Autodesk Fusion 360 part; units mm, degrees
(part 4 of 4)
extrude "Extrusão23" cut sketch "Esboço21" against normal blind 1 contours S0 S1 S2 S3 L28 L29 S4 L30 L31 S5 S6 S7 S8 S9 S10 S11 S12 S13 S14 S15 S16 S17 S18 L32 L33 S19 L34 L35 S20 S21 S22 S23 S24 S25 S26 S27 S28 S29 S30 S31 S32 S33 S34 S35 S36 L36 L37 S37 S38 S39 S40 S41 S42 S43 S44 S45 S46 S47 S48 S49 S50 S51 S52 S53 S54 S55 S56 S57 S58 S59 S60 S61 S62 S63 S64 S65 S66 S67 S68 S69 L38 L39 S70 S71 S72 S73 S74 S75 S76 S77 S78 S79 S80 S81 S82 L40 L41 S83 S84 S85 L42 L43 S86 S87 S88 S89 S90 S91 S92 S93 L44 L45 S94 L46 L47 S95 S96 S97 S98 S99 S100 L48 L49 S101 S102 S103 S104 S105 S106 S107 | S248 S249 S250 S251 S252 S253 S254 S255 S256 S257 S258 S259 S260 S261 S262 S263 S264 S265 S266 S267 S268 S269 S270 S271 S272 S273 S274 S275 S276 S277 S278 S279 S280 S281 S282 S283 S284 S285 S286 S287 S288 S289 S290 S291 S292 | S311 S312 S313 S314 S315 S316 S317 | S324 S325 S326 S327 S328 S329 S330 S331 S332 S333 S334 S335 S336 S337 L62 L63 S338 S339 S340 S341 S342 S343 S344 S345 S346 S347 S348 S349 S350 S351 S352 S353 S354 S355 S356 S357 S358 S359 S360 S361 S362 S363 S364 S365 S366 S367 S368 S369 S370 S371 L64 L65 S372 S373 L66 L67 S374 S375 S376 S377 S378 S379 S380 S381 S382 S383 S384 S385 S386 L68 L69 S387 L70 L71 S388 S389 S390 S391 S392 S393 S394 S395 S396 S397 S398 S399 S400 S401 S402 S403 S404 S405 S406 S407 S408 S409 S410 S411 S412 S413 S414 L72 L73 S415 S416 S417 S418 S419 S420 S421 S422 S423 S424 S425 S426 L74 L75 S427 S428 S429 S430 S431 S432 S433 S434 S435 S436 | S654 S655 S656 | S672 S673 S674 S675 S676 S677 L100 L101 L102 L103 S678 bodies 2
sketch "Esboço22" plane through (0, 0, 24.51) normal (0, 0, -1) x (1, 0, 0)
  spline S0 degree 3 poles (210.2876, 111.6079) (210.4619, 111.38) (210.6257, 111.1299) (210.7764, 110.864) knots 0 0 0 0 0.232069 0.232069 0.232069 0.232069
  line L0 (210.7764, 110.864) -> (215.399, 110.864)
  line L1 (215.399, 110.864) -> (215.399, 125.864)
  line L2 (215.399, 125.864) -> (200.399, 125.864)
  line L3 (200.399, 125.864) -> (200.399, 112.7841)
  spline S1 degree 3 poles (200.399, 112.7841) (201.1419, 113.2879) (202.0331, 113.7075) (202.8355, 113.9186) knots 0.268953 0.268953 0.268953 0.268953 1 1 1 1
  spline S2 degree 3 poles (202.8355, 113.9186) (203.0738, 113.9836) (203.6226, 114.0703) (204.0631, 114.1136) knots 0 0 0 0 1 1 1 1
  spline S3 degree 3 poles (204.0631, 114.1136) (206.5038, 114.3663) (208.93, 113.3915) (210.2876, 111.6079) knots 0 0 0 0 1 1 1 1
  circle A0 centre (207.899, 118.364) radius 2.5
  line L4 (215.399, 121.8438) -> (200.399, 121.8438)
  line L5 (200.399, 121.8438) -> (200.399, 114.8842)
  line L6 (200.399, 114.8842) -> (215.399, 114.8842)
  line L7 (215.399, 114.8842) -> (215.399, 121.8438)
  line L8 (215.399, 121.8438) -> (200.399, 114.8842) construction
  line L9 (200.399, 121.8438) -> (215.399, 114.8842) construction
  line L10 (200.399, 114.8842) -> (215.399, 114.8842)
  line L11 (215.399, 114.8842) -> (215.399, 110.864)
  line L12 (215.399, 110.864) -> (200.399, 110.864)
  line L13 (200.399, 110.864) -> (200.399, 114.8842)
  point P0 (207.899, 118.364)
  constraint horizontal L4
  constraint perpendicular L4 L5
  constraint parallel L4 L6
  constraint parallel L5 L7
  constraint coincident L8 P0
  constraint coincident L9 P0
  constraint coincident L1 L4.start
  constraint coincident P0 A0.centre
  constraint horizontal L10
  constraint vertical L11
  constraint horizontal L12
  constraint vertical L13
  constraint coincident L0.end L1.start
extrude "Extrusão24" add sketch "Esboço22" along normal blind 1 contours S0 L0 L1 L3 S1 S2 S3 L6 L10 L11 L12 L13 | S0 S1 S2 S3 L12 L13 | L1 L2 L3 L4 bodies 2
sketch "Esboço23" plane through (269, 0, 0) normal (1, 0, 0) x (0, 1, 0)
  line L0 (-40.5, 23.51) -> (-140.5, 23.51)
  line L1 (-140.5, 23.51) -> (-140.5, 13.51)
  line L2 (-140.5, 13.51) -> (-40.5, 13.51)
  line L3 (-40.5, 13.51) -> (-40.5, 23.51)
  line L4 (-40.5, 23.51) -> (-51.0189, 13.51)
  constraint coincident L0.start L3.end
  constraint coincident L2 L4.end
extrude "Extrusão25" cut sketch "Esboço23" against normal blind 185 contours L2 L3 L4 bodies 2
sketch "Esboço24" plane through (271.5, 0, 0) normal (1, 0, 0) x (0, 1, 0)
  circle A0 centre (-90.5, 11.01) radius 7
  line L0 (-38, -11.49) -> (-38, 23.51)
  line L1 (-38, 23.51) -> (-143, 23.51)
  line L2 (-143, 23.51) -> (-143, -11.49)
  line L3 (-143, -11.49) -> (-38, -11.49)
  line L4 (-60.626, 6.295) -> (-60.226, 6.295)
  line L5 (-60.226, 6.295) -> (-73.226, 6.295)
  line L6 (-73.226, 6.295) -> (-73.226, 13.295)
  line L7 (-73.226, 13.295) -> (-60.226, 13.295)
  line L8 (-60.226, 13.295) -> (-60.226, 6.295)
  dimension "d90" = 13
  dimension "d91" = 7
  constraint horizontal L5
  constraint vertical L6
  constraint horizontal L7
  constraint vertical L8
  constraint coincident L4.end L5.start
  measures "d90" distance of L4.end L5.end
  measures "d91" distance of L4.end L7.end
extrude "Extrusão26" cut sketch "Esboço24" against normal blind 14 contours L4 L5 L6 L7 L8 bodies 1
sketch "Esboço25" plane through (0, -99, 0) normal (0, -1, 0) x (1, 0, 0)
  line L0 (159.5, 19.5) -> (166.5, 19.5)
  line L1 (166.5, 19.5) -> (166.5, 21.5)
  line L2 (166.5, 21.5) -> (157.5, 21.5)
  line L3 (157.5, 21.5) -> (157.5, 0.5)
  line L4 (157.5, 0.5) -> (166.5, 0.5)
  line L5 (166.5, 0.5) -> (166.5, 2.5)
  line L6 (166.5, 2.5) -> (159.5, 2.5)
  line L7 (159.5, 2.5) -> (159.5, 19.5)
  line L8 (159.5, 11) -> (157.5, 11)
  constraint midpoint L7 L8.start
  constraint midpoint L3 L8.end
extrude "Extrusão27" add sketch "Esboço25" along normal blind 44 contours L0 L1 L2 L3 L7 L8 bodies 1 7
sketch "Esboço26" plane through (0, -143, 0) normal (0, -1, 0) x (1, 0, 0)
  line L0 (271.5, -11.49) -> (271.5, 23.51)
  line L1 (271.5, 23.51) -> (166.5, 23.51)
  line L2 (166.5, 23.51) -> (166.5, 21.5)
  line L3 (166.5, 21.5) -> (157.5, 21.5)
  line L4 (157.5, 21.5) -> (157.5, 11)
  line L5 (157.5, 11) -> (159.5, 11)
  line L6 (159.5, 11) -> (159.5, 19.5)
  line L7 (159.5, 19.5) -> (166.5, 19.5)
  line L8 (166.5, 19.5) -> (166.5, -11.49)
  line L9 (166.5, -11.49) -> (271.5, -11.49)
  line L10 (157.5, 21.5) -> (166.5, 21.5)
  line L11 (166.5, 21.5) -> (166.5, 11)
  line L12 (166.5, 11) -> (157.5, 11)
  line L13 (157.5, 11) -> (157.5, 21.5)
  constraint horizontal L10
  constraint vertical L11
  constraint horizontal L12
  constraint vertical L13
  constraint coincident L8 L11.end
  constraint coincident L3.end L4.start
extrude "Extrusão28" add sketch "Esboço26" against normal blind 2 contours L6 L7 L8 L11 L12 bodies 1
sketch "Esboço27" plane through (0, -75, 0) normal (0, 1, 0) x (-1, 0, 0)
  line L0 (-166.5, 21.5) -> (-166.5, 0.5)
  line L1 (-166.5, 0.5) -> (-157.5, 0.5)
  line L2 (-157.5, 0.5) -> (-157.5, 21.5)
  line L3 (-157.5, 21.5) -> (-166.5, 21.5)
  line L4 (-160, 19) -> (-164, 19)
  line L5 (-164, 19) -> (-164, 3)
  line L6 (-164, 3) -> (-160, 3)
  line L7 (-160, 3) -> (-160, 19)
  line L8 (-160, 19) -> (-164, 3) construction
  line L9 (-164, 19) -> (-160, 3) construction
  point P0 (-162, 11)
  constraint horizontal L4
  constraint perpendicular L4 L5
  constraint parallel L4 L6
  constraint parallel L5 L7
  constraint coincident L8 P0
  constraint coincident L9 P0
extrude "Extrusão29" cut sketch "Esboço27" against normal blind 7 contours L4 L5 L6 L7 bodies 1
sketch "Esboço28" plane through (271.5, 0, 0) normal (1, 0, 0) x (0, 1, 0)
  line L0 (-73.226, 6.295) -> (-73.226, 13.295)
  line L1 (-73.226, 13.295) -> (-60.226, 13.295)
  line L2 (-60.226, 13.295) -> (-60.226, 6.295)
  line L3 (-60.226, 6.295) -> (-73.226, 6.295)
  circle A0 centre (-90.5, 11.01) radius 7
  line L4 (-38, -11.49) -> (-38, 23.51)
  line L5 (-38, 23.51) -> (-143, 23.51)
  line L6 (-143, 23.51) -> (-143, -11.49)
  line L7 (-143, -11.49) -> (-38, -11.49)
  line L8 (-57.226, 3.295) -> (-76.226, 3.295)
  line L9 (-76.226, 3.295) -> (-76.226, 16.295)
  line L10 (-76.226, 16.295) -> (-57.226, 16.295)
  line L11 (-57.226, 16.295) -> (-57.226, 3.295)
  dimension "d100" = -3
extrude "Extrusão30" add sketch "Esboço28" along normal blind 3 contours L8 L9 L10 L11 bodies 1
sketch "Esboço29" plane through (0, -57.226, 0) normal (0, 1, 0) x (-1, 0, 0)
  line L0 (-271.5, 3.295) -> (-271.5, 16.295)
  line L1 (-271.5, 16.295) -> (-274.5, 16.295)
  line L2 (-274.5, 16.295) -> (-274.5, 3.295)
  line L3 (-274.5, 3.295) -> (-271.5, 3.295)
  line L4 (-274.5, 5.5) -> (-271.5, 3.295)
  point P0 (-274.5, 6.295)
  constraint coincident L2 L4.start
  constraint coincident L0.start L3.end
extrude "Extrusão31" cut sketch "Esboço29" against normal blind 24 contours L2 L3 L4 bodies 1
extrude "Extrusão32" add 1 faces at (162.6667, -75.6667, 3) along direction (0, 0, 1) blind 16 on bodies 1 bodies 1
extrude "Extrusão33" add 5 faces at (214.0299, -82.9846, 24.51) (177.4969, -77.5992, 24.51) (211.0301, -69.4647, 24.51) (186.2063, -114.4199, 24.51) (198.407, -103.7815, 24.51) along direction (0, 0, 1) blind 1 on bodies 2 bodies 2
extrude "Extrusão34" add 1 faces at (188.6509, -105.5317, 24.51) along direction (0, 0, 1) blind 1 on bodies 2 bodies 2
sketch "Esboço30" plane through (0, 0, 25.51) normal (0, 0, 1) x (-1, 0, 0)
  line L0 (-234.4628, 67.952) -> (-232.5162, 67.952)
  spline S0 degree 3 poles (-232.5162, 67.952) (-232.3484, 67.8486) (-232.1846, 67.7473) (-232.022, 67.6464) knots -0.55439 -0.55439 -0.55439 -0.55439 -0.461759 -0.461759 -0.461759 -0.461759
  line L1 (-232.022, 67.6464) -> (-232.022, 66.4454)
  spline S1 degree 3 poles (-232.022, 66.4454) (-232.8883, 66.9868) (-233.7468, 67.5194) (-234.247, 67.8195) knots -0.659701 -0.659701 -0.659701 -0.659701 0 0 0 0
  spline S2 degree 3 poles (-234.247, 67.8195) (-234.3097, 67.8581) (-234.382, 67.9025) (-234.4628, 67.952) knots -1 -1 -1 -1 -0.916474 -0.916474 -0.916474 -0.916474
  arc A0 (-264.8266, 72.716) -> (-256.8894, 72.716) centre (-260.858, 77.216) ccw
  line L2 (-264.8266, 72.716) -> (-256.8894, 72.716)
  arc A1 (-203.4723, 131.348) -> (-203.0106, 132.848) centre (-208.9267, 133.848) ccw
  line L3 (-203.4723, 131.348) -> (-214.381, 131.348)
  arc A2 (-214.8427, 132.848) -> (-214.381, 131.348) centre (-208.9267, 133.848) ccw
  line L4 (-214.8427, 132.848) -> (-203.0106, 132.848)
  arc A3 (-212.8953, 129.348) -> (-204.958, 129.348) centre (-208.9267, 133.848) ccw
  line L5 (-212.8953, 129.348) -> (-204.958, 129.348)
  line L6 (-255.4036, 74.716) -> (-266.3124, 74.716)
  arc A4 (-266.7741, 76.216) -> (-266.3124, 74.716) centre (-260.858, 77.216) ccw
  line L7 (-266.7741, 76.216) -> (-254.9419, 76.216)
  arc A5 (-255.4036, 74.716) -> (-254.9419, 76.216) centre (-260.858, 77.216) ccw
  line L8 (-203.0106, 134.848) -> (-214.8427, 134.848)
  arc A6 (-214.381, 136.348) -> (-214.8427, 134.848) centre (-208.9267, 133.848) ccw
  line L9 (-214.381, 136.348) -> (-203.4723, 136.348)
  arc A7 (-203.0106, 134.848) -> (-203.4723, 136.348) centre (-208.9267, 133.848) ccw
  line L10 (-254.9419, 78.216) -> (-266.7741, 78.216)
  arc A8 (-266.3124, 79.716) -> (-266.7741, 78.216) centre (-260.858, 77.216) ccw
  line L11 (-266.3124, 79.716) -> (-255.4036, 79.716)
  arc A9 (-254.9419, 78.216) -> (-255.4036, 79.716) centre (-260.858, 77.216) ccw
  circle A10 centre (-239.522, 60.452) radius 2.5
  circle A11 centre (-207.899, 118.364) radius 2.5
  line L12 (-257.756, 60.626) -> (-257.806, 60.626)
  line L13 (-257.806, 60.626) -> (-257.806, 60.226)
  line L14 (-257.806, 60.226) -> (-265.506, 60.226)
  line L15 (-265.506, 60.226) -> (-265.506, 60.626)
  line L16 (-265.506, 60.626) -> (-265.556, 60.626)
  line L17 (-265.556, 60.626) -> (-265.556, 63.326)
  line L18 (-265.556, 63.326) -> (-265.506, 63.326)
  line L19 (-265.506, 63.326) -> (-265.506, 63.726)
  line L20 (-265.506, 63.726) -> (-257.806, 63.726)
  line L21 (-257.806, 63.726) -> (-257.806, 63.326)
  line L22 (-257.806, 63.326) -> (-257.756, 63.326)
  line L23 (-257.756, 63.326) -> (-257.756, 60.626)
  line L24 (-204.958, 138.348) -> (-212.8953, 138.348)
  arc A12 (-204.958, 138.348) -> (-212.8953, 138.348) centre (-208.9267, 133.848) ccw
  line L25 (-256.8894, 81.716) -> (-264.8266, 81.716)
  arc A13 (-256.8894, 81.716) -> (-264.8266, 81.716) centre (-260.858, 77.216) ccw
  line L26 (-271.5, 38) -> (-166.5, 38)
  line L27 (-166.5, 38) -> (-166.5, 143)
  line L28 (-166.5, 143) -> (-271.5, 143)
  line L29 (-271.5, 143) -> (-271.5, 38)
extrude "Extrusão35" add sketch "Esboço30" against normal blind 2 contours L12 L13 L14 L15 L16 L17 L18 L19 L20 L21 L22 L23 bodies 2
sketch "Esboço31" plane through (0, 0, 25.51) normal (0, 0, 1) x (-1, 0, 0)
  line L0 (-234.4628, 67.952) -> (-232.5162, 67.952)
  spline S0 degree 3 poles (-232.5162, 67.952) (-232.3484, 67.8486) (-232.1846, 67.7473) (-232.022, 67.6464) knots -0.55439 -0.55439 -0.55439 -0.55439 -0.461759 -0.461759 -0.461759 -0.461759
  line L1 (-232.022, 67.6464) -> (-232.022, 66.4454)
  spline S1 degree 3 poles (-232.022, 66.4454) (-232.8883, 66.9868) (-233.7468, 67.5194) (-234.247, 67.8195) knots -0.659701 -0.659701 -0.659701 -0.659701 0 0 0 0
  spline S2 degree 3 poles (-234.247, 67.8195) (-234.3097, 67.8581) (-234.382, 67.9025) (-234.4628, 67.952) knots -1 -1 -1 -1 -0.916474 -0.916474 -0.916474 -0.916474
  arc A0 (-264.8266, 72.716) -> (-256.8894, 72.716) centre (-260.858, 77.216) ccw
  line L2 (-264.8266, 72.716) -> (-256.8894, 72.716)
  arc A1 (-203.4723, 131.348) -> (-203.0106, 132.848) centre (-208.9267, 133.848) ccw
  line L3 (-203.4723, 131.348) -> (-214.381, 131.348)
  arc A2 (-214.8427, 132.848) -> (-214.381, 131.348) centre (-208.9267, 133.848) ccw
  line L4 (-214.8427, 132.848) -> (-203.0106, 132.848)
  arc A3 (-212.8953, 129.348) -> (-204.958, 129.348) centre (-208.9267, 133.848) ccw
  line L5 (-212.8953, 129.348) -> (-204.958, 129.348)
  line L6 (-255.4036, 74.716) -> (-266.3124, 74.716)
  arc A4 (-266.7741, 76.216) -> (-266.3124, 74.716) centre (-260.858, 77.216) ccw
  line L7 (-266.7741, 76.216) -> (-254.9419, 76.216)
  arc A5 (-255.4036, 74.716) -> (-254.9419, 76.216) centre (-260.858, 77.216) ccw
  line L8 (-203.0106, 134.848) -> (-214.8427, 134.848)
  arc A6 (-214.381, 136.348) -> (-214.8427, 134.848) centre (-208.9267, 133.848) ccw
  line L9 (-214.381, 136.348) -> (-203.4723, 136.348)
  arc A7 (-203.0106, 134.848) -> (-203.4723, 136.348) centre (-208.9267, 133.848) ccw
  line L10 (-254.9419, 78.216) -> (-266.7741, 78.216)
  arc A8 (-266.3124, 79.716) -> (-266.7741, 78.216) centre (-260.858, 77.216) ccw
  line L11 (-266.3124, 79.716) -> (-255.4036, 79.716)
  arc A9 (-254.9419, 78.216) -> (-255.4036, 79.716) centre (-260.858, 77.216) ccw
  circle A10 centre (-239.522, 60.452) radius 2.5
  circle A11 centre (-207.899, 118.364) radius 2.5
  line L12 (-204.958, 138.348) -> (-212.8953, 138.348)
  arc A12 (-204.958, 138.348) -> (-212.8953, 138.348) centre (-208.9267, 133.848) ccw
  line L13 (-256.8894, 81.716) -> (-264.8266, 81.716)
  arc A13 (-256.8894, 81.716) -> (-264.8266, 81.716) centre (-260.858, 77.216) ccw
  line L14 (-271.5, 38) -> (-166.5, 38)
  line L15 (-166.5, 38) -> (-166.5, 143)
  line L16 (-166.5, 143) -> (-271.5, 143)
  line L17 (-271.5, 143) -> (-271.5, 38)
extrude "Extrusão36" add sketch "Esboço31" against normal blind 1 contours L0 S0 L1 S1 S2 bodies 2
sketch "Esboço32" plane through (166.5, 0, 0) normal (-1, 0, 0) x (0, -1, 0)
  line L0 (38, 23.51) -> (143, 23.51)
  line L1 (143, 23.51) -> (143, 25.51)
  line L2 (143, 25.51) -> (38, 25.51)
  line L3 (38, 25.51) -> (38, 23.51)
  line L4 (143, 25.51) -> (150, 25.51)
  circle A0 centre (146.5, 23.2422) radius 1
  line L5 (143, 25.51) -> (150, 25.51)
  line L6 (150, 25.51) -> (150, 21.01)
  line L7 (150, 21.01) -> (143, 21.01)
  line L8 (143, 21.01) -> (143, 25.51)
  dimension "d115" = 2
  dimension "d116" = 4.5
  constraint coincident L1.end L2.start
  constraint perpendicular L1 L4
  constraint horizontal L5
  constraint vertical L6
  constraint horizontal L7
  constraint vertical L8
  measures "d115" diameter of A0
  measures "d116" distance of L1.end L7.end
sketch "Esboço33" plane through (271.5, 0, 0) normal (1, 0, 0) x (0, 1, 0)
  line L0 (-57.226, 16.295) -> (-57.226, 3.295)
  line L1 (-57.226, 3.295) -> (-76.226, 3.295)
  line L2 (-76.226, 3.295) -> (-76.226, 16.295)
  line L3 (-76.226, 16.295) -> (-57.226, 16.295)
  circle A0 centre (-90.5, 11.01) radius 7
  line L4 (-38, -11.49) -> (-38, 23.51)
  line L5 (-38, 23.51) -> (-143, 23.51)
  line L6 (-143, 23.51) -> (-143, -11.49)
  line L7 (-143, -11.49) -> (-38, -11.49)
extrude "Extrusão38" cut sketch "Esboço33" against normal blind 29 contours A0 bodies 2
sketch "Esboço34" plane through (169, 0, 0) normal (-1, 0, 0) x (0, -1, 0)
  line L0 (40.5, 23.51) -> (51.0189, 13.51)
  line L1 (51.0189, 13.51) -> (83.9617, 13.51)
  arc A0 (97.0383, 13.51) -> (83.9617, 13.51) centre (90.5, 11.01) ccw
  line L2 (97.0383, 13.51) -> (140.5, 13.51)
  line L3 (140.5, 13.51) -> (140.5, 23.51)
  line L4 (140.5, 23.51) -> (40.5, 23.51)
  line L5 (83.9617, 13.51) -> (97.0383, 13.51)
  constraint coincident L1.end A0.end
  constraint coincident A0.start L2.start
extrude "Extrusão39" add sketch "Esboço34" against normal blind 1.5 contours A0 L5 bodies 2
hidden bodies 3 4 5 6
equation "d24 = -d23"
named bodies: "case", "tampa", "dobradiça_C", "dobradiça_B", "dobradiça_B (1)", "dobradiça_C (1)", "GPS_suporte"
